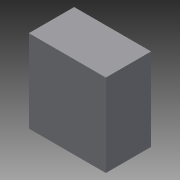
# Autodesk Inventor part: small24v2600mahbattery
Saved by Autodesk Inventor 2015 (Build 190159000, 159)
## iProperties
Created: 2014-09-28
Part Number: small24v2600mahbattery
Material: Generic
Document SubType Name: Modeling
Designer: ericd_000
Density: 1 g/cm^3
Appearance: Default
Author: ericd_000
Autodesk Inventor part; units mm, degrees
ref_plane "YZ Plane" through (0, 0, 0) normal (1, 0, 0) x (0, 1, 0)
ref_plane "XZ Plane" through (0, 0, 0) normal (0, 1, 0) x (-1, 0, 0)
ref_plane "XY Plane" through (0, 0, 0) normal (0, 0, 1) x (1, 0, 0)
sketch "Sketch1" plane through (0, 0, 0) normal (0, 1, 0) x (-1, 0, 0)
  line L0 (18.931, 39.3601) -> (-49.069, 39.3601)
  line L1 (-49.069, 39.3601) -> (-49.069, -33.6399)
  line L2 (-49.069, -33.6399) -> (18.931, -33.6399)
  line L3 (18.931, -33.6399) -> (18.931, 39.3601)
  point P0 (0, 0)
  dimension "d0" = 73
  dimension "d1" = 68
  constraints: 8 end point, 2 parallel, 1 horizontal, 1 perpendicular
  measures "d0" distance of L2.end L0.start
  measures "d1" distance of L0.start L0.end
extrude "Extrusion1" add sketch "Sketch1" along normal blind 40
body "Solid1"
